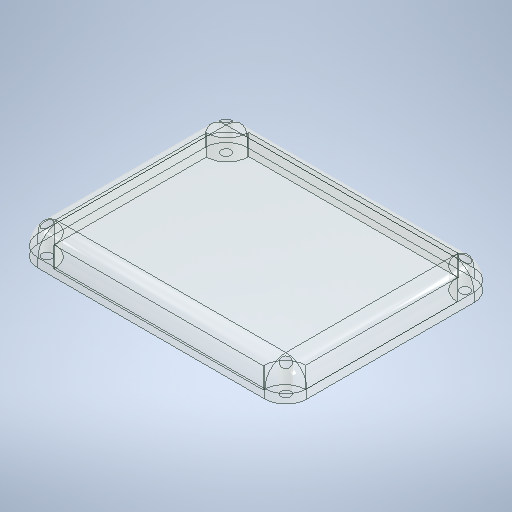
# Autodesk Inventor part: acrilico
Saved by Autodesk Inventor 2025 (Build 290162000, 162)
## iProperties
Created: 2024-05-01
Part Number: acrilico
Material: Glass
Document SubType Name: Modeling
Designer: kaike
Density: 2.18 g/cm^3
Appearance: Clear
Mass: 48.3718 g
Surface Area: 170.401 cm^2
Volume: 22.1889 cm^3
Author: kaike
Autodesk Inventor part; units mm, degrees
ref_plane "YZ Plane" through (0, 0, 0) normal (1, 0, 0) x (0, 1, 0)
ref_plane "XZ Plane" through (0, 0, 0) normal (0, 1, 0) x (-1, 0, 0)
ref_plane "XY Plane" through (0, 0, 0) normal (0, 0, 1) x (1, 0, 0)
sketch "Sketch1" plane through (0, 0, 0) normal (0, 1, 0) x (-1, 0, 0)
  line L0 (0, 0) -> (90, 0)
  line L1 (90, 0) -> (90, -70)
  line L2 (90, -70) -> (0, -70)
  line L3 (0, -70) -> (0, 0)
  line L4 (0, 0) -> (0, -5)
  circle A0 centre (5, -5) radius 1.6095
  circle A1 centre (5, -65) radius 1.6095
  circle A2 centre (85, -5) radius 1.6095
  circle A3 centre (85, -65) radius 1.6095
  dimension "d0" = 90
  dimension "d1" = 70
  dimension "d5" = 3.219
  constraints: 10 end point, 4 centre point, 3 perpendicular, 1 horizontal
  measures "d0" distance of L0.start L0.end
  measures "d1" distance of L0.end L1.end
  measures "d5" diameter of A0
extrude "Extrusion1" add sketch "Sketch1" along normal blind 10
sketch "Sketch2" plane through (0, 0, 0) normal (0, -1, 0) x (1, 0, 0)
  line L0 (-3, -60.3846) -> (-87, -60.3846)
  line L1 (-3, -9.614) -> (-3, -60.3846)
  line L2 (-3, -9.614) -> (-87, -9.614)
  line L3 (-87, -60.3846) -> (-87, -9.614)
  constraints: 8 end point, 2 vertical, 1 horizontal
extrude "Extrusion2" cut sketch "Sketch2" against normal blind 7
sketch "Sketch3" plane through (0, 0, 0) normal (0, -1, 0) x (1, 0, 0)
  line L0 (-45, -2.3836) -> (-9.9317, -2.3836)
  line L1 (-9.9317, -2.3836) -> (-9.9317, -9.5344)
  line L2 (-45, -2.3836) -> (-80.0683, -2.3836)
  line L3 (-80.0683, -2.3836) -> (-80.0683, -9.5344)
  line L4 (-45, -67.615) -> (-9.9317, -67.615)
  line L5 (-9.9317, -67.615) -> (-9.9317, -60.4642)
  line L6 (-45, -67.615) -> (-80.0683, -67.615)
  line L7 (-80.0683, -67.615) -> (-80.0683, -60.4642)
  line L8 (-80.0683, -60.4642) -> (-80.0683, -9.5344)
  line L9 (-9.9317, -60.4642) -> (-9.9317, -9.5344)
  point P0 (0, 0)
  point P1 (-5, -5)
  dimension "d15" = 4.9317
  dimension "d17" = 65.2314
  dimension "d18" = 70.1366
  constraints: 20 end point, 2 vertical, 1 horizontal, 1 perpendicular
  measures "d15" horizontal distance of L0.end point (-5, -5)
  measures "d17" distance of L2.end L6.end
  measures "d18" distance of L6.end L4.end
extrude "Extrusion3" cut sketch "Sketch3" against normal blind 7
fillet "Fillet2" radius 7 2 edges at (-90, 10, -35) (0, 10, -35)
fillet "Fillet3" radius 7 10 edges at (-87.9497, 7.9497, -70) (-90, 1.5, -70) (-2.0503, 7.9497, -70) (0, 1.5, -70) (-45, 10, -70) (-2.0503, 7.9497, 0) (0, 1.5, 0) (-87.9497, 7.9497, 0) (-90, 1.5, 0) (-45, 10, 0)
fillet "Fillet4" radius 7 4 edges at (-80.0683, 3.5, -9.614) (-80.0683, 3.5, -60.3846) (-9.9317, 3.5, -60.3846) (-9.9317, 3.5, -9.614)
body "Solid1"
